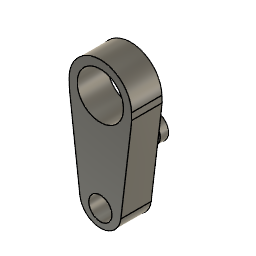
LEG DESIGN 2 (Autodesk Fusion 360 design; units mm, degrees)
part number: 2026-03-06-04-06-48-777
Autodesk Fusion 360 part; units mm, degrees
sketch "Sketch1" plane through (0, 0, 0) normal (0, 1, 0) x (1, 0, 0)
  line L0 (36.8758, -36.9029) -> (23.6155, 73.0203)
  circle A0 centre (-1.2046, -43.7212) radius 28
  line L1 (-38.7425, -32.3133) -> (-39.0485, -42.5947)
  circle A1 centre (-1.2046, 74.3196) radius 14
  arc A2 (23.6155, 73.0203) -> (13.7954, 90.0262) centre (-1.2046, 70.0262) ccw
  arc A3 (13.7954, 90.0262) -> (-26.0243, 73.0229) centre (-1.2046, 70.0262) ccw
  line L2 (36.6393, -44.8476) -> (36.8758, -36.9029)
  line L3 (-38.7425, -32.3133) -> (-26.0243, 73.0229)
  arc A4 (-39.0485, -42.5947) -> (36.6393, -44.8476) centre (-1.2046, -43.7212) ccw
  dimension "d1" = 28
  dimension "d2" = 25
  dimension "d3" = 25
  dimension "d4" = 105.3362
  constraint parallel L1 L2
  constraint tangent L1 A4
  constraint tangent L2 A4
  constraint concentric A0 A4
  constraint tangent L0 A2
  constraint tangent A3 L3
  constraint tangent A2 A3
  measures "d1" diameter of A1
  measures "d2" radius of A2
  measures "d3" radius of A3
  measures "d4" vertical distance of L1.start A3.end
extrude "Extrude1" add sketch "Sketch1" along normal blind 0.36
extrude "Extrude2" add 1 faces at (-27.8097, 0, -6.2933) along direction (0, -1, 0) blind 36.4
sketch "Sketch2" plane through (0, 0.36, 0) normal (0, 1, 0) x (-1, 0, 0)
  circle A0 centre (1.2046, -74.3196) radius 14
  circle A1 centre (1.2046, 43.7212) radius 28
  line L0 (38.7425, 32.3133) -> (39.0485, 42.5947)
  arc A2 (39.0485, 42.5947) -> (-36.6393, 44.8476) centre (1.2046, 43.7212) ccw
  line L1 (-36.6393, 44.8476) -> (-36.8758, 36.9029)
  line L2 (-36.8758, 36.9029) -> (-23.6155, -73.0203)
  arc A3 (-23.6155, -73.0203) -> (26.0243, -73.0229) centre (1.2046, -70.0262) ccw
  line L3 (26.0243, -73.0229) -> (38.7425, 32.3133)
  circle A4 centre (0.422, -20.3548) radius 10
  dimension "d9" = 20
  measures "d9" diameter of A4
extrude "Extrude3" add sketch "Sketch2" along normal blind 20 contours A4
sketch "Sketch3" plane through (0, 20.36, 0) normal (0, 1, 0) x (-1, 0, 0)
  circle A0 centre (0.422, -20.3548) radius 10
  circle A1 centre (0.422, -20.3548) radius 15
  dimension "d12" = 30
  constraint concentric A0 A1
  measures "d12" diameter of A1
extrude "Extrude4" add sketch "Sketch3" along normal blind 10 contours A0 | A1
